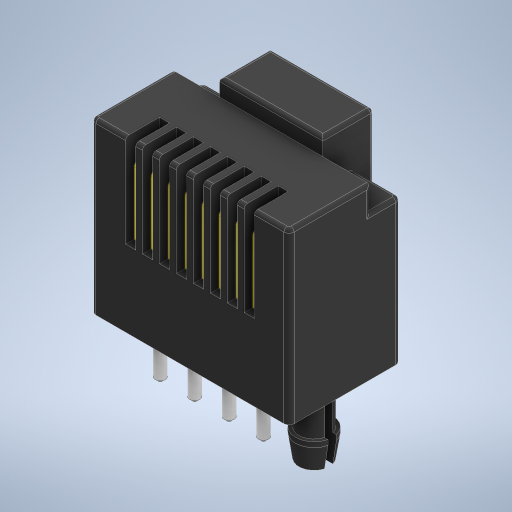
# Autodesk Inventor part: KINSUN AJP92A8813
Saved by Autodesk Inventor 2024 (Build 280153000, 153)
## iProperties
Created: 2026-08-25
Part Number: KINSUN AJP92A8813
Material: Generic
Document SubType Name: Modeling
Designer: murashkindv
Density: 1 g/cm^3
Appearance: Default
Author: murashkindv
Autodesk Inventor part; units mm, degrees
ref_plane "YZ Plane" through (0, 0, 0) normal (1, 0, 0) x (0, 1, 0)
ref_plane "XZ Plane" through (0, 0, 0) normal (0, 1, 0) x (-1, 0, 0)
ref_plane "XY Plane" through (0, 0, 0) normal (0, 0, 1) x (1, 0, 0)
sketch "Sketch6" plane through (0, 0, 0) normal (0, 1, 0) x (-1, 0, 0)
  circle A0 centre (-4.89, 0.635) radius 1.1
  circle A1 centre (4.89, -1.27) radius 1.1
  line L0 (4.89, -1.27) -> (-4.89, 0.635) construction
  line L1 (3.048, 0) -> (0, 0) construction
  line L2 (5.99, -1.52) -> (3.79, -1.52)
  line L3 (3.79, -1.52) -> (3.79, -1.02) construction
  line L4 (3.79, -1.02) -> (5.99, -1.02)
  line L5 (5.99, -1.02) -> (5.99, -1.52) construction
  line L6 (5.99, -1.52) -> (3.79, -1.02) construction
  line L7 (3.79, -1.52) -> (5.99, -1.02) construction
  line L8 (-5.99, 0.385) -> (-3.79, 0.385)
  line L9 (-3.79, 0.385) -> (-3.79, 0.885) construction
  line L10 (-3.79, 0.885) -> (-5.99, 0.885)
  line L11 (-5.99, 0.885) -> (-5.99, 0.385) construction
  line L12 (-5.99, 0.385) -> (-3.79, 0.885) construction
  line L13 (-3.79, 0.385) -> (-5.99, 0.885) construction
  point P0 (0, -0.3175)
  point P1 (-3.79, 0.635)
  point P2 (-4.64, -0.4362)
  point P3 (-5.14, -0.4362)
  point P4 (-5.99, 0.635)
  point P5 (3.79, -1.27)
  point P6 (4.64, -0.1988)
  point P7 (5.99, -1.27)
  point P8 (5.14, -2.3412)
  point P9 (-5.9612, 0.885)
  point P10 (-3.8188, 0.885)
  point P11 (-5.9612, 0.385)
  point P12 (-3.8188, 0.385)
  point P13 (5.9612, -1.02)
  point P14 (5.9612, -1.52)
  point P15 (3.8188, -1.02)
  point P16 (3.8188, -1.52)
  dimension "d77" = 2.2
  dimension "d78" = 9.78
  dimension "d89" = 1.27
  dimension "d90" = 0.635
  dimension "d160" = 0.5
  constraints: 28 end point, 6 parallel, 5 midpoint, 3 horizontal, 2 centre point, 2 perpendicular, 1 coincident, 1 equal radius, 1 horizontal alignment, 1 tangent, 1 vertical alignment, 1 other
  measures "d77" diameter of A1
  measures "d78" horizontal distance of L0.end L0.start
  measures "d89" vertical distance of L1.end L0.start
  measures "d90" vertical distance of L1.end L0.end
  measures "d160" distance between parallel lines of L2 L4
sketch "Sketch7" plane through (0, 0, 0) normal (0, 1, 0) x (-1, 0, 0)
  circle A0 centre (2.54, -1.27) radius 0.3
  circle A1 centre (3.556, 1.27) radius 0.3
  line L0 (2.54, -1.27) -> (3.556, 1.27) construction
  line L1 (3.048, 0) -> (0, 0) construction
  circle A2 centre (0.508, -1.27) radius 0.3
  circle A3 centre (1.524, 1.27) radius 0.3
  circle A4 centre (-1.524, -1.27) radius 0.3
  circle A5 centre (-0.508, 1.27) radius 0.3
  circle A6 centre (-3.556, -1.27) radius 0.3
  circle A7 centre (-2.54, 1.27) radius 0.3
  line L2 (-2.54, 1.27) -> (2.54, -1.27) construction
  dimension "d95" = 0.6
  dimension "d97" = 1.016
  dimension "d98" = 2.032
  dimension "d99" = 7.112
  dimension "d101" = 1.27
  constraints: 8 centre point, 6 end point, 2 horizontal, 2 midpoint, 1 coincident, 1 equal radius, 1 horizontal alignment, 12 other
  measures "d95" diameter of A0
  measures "d97" horizontal distance of L0.end L2.end
  measures "d98" distance of L2.end A2.centre
  measures "d99" horizontal distance of A6.centre L0.end
  measures "d101" vertical distance of point (0, 0) L2.end
sketch "Sketch8" plane through (0, 0, 0) normal (0, 1, 0) x (-1, 0, 0)
  line L0 (5.55, -3.525) -> (-5.55, -3.525)
  line L1 (-5.85, -3.225) -> (-5.85, 2.775)
  line L2 (-5.55, 3.075) -> (5.55, 3.075)
  line L3 (5.85, 2.775) -> (5.85, -3.225)
  arc A0 (5.55, -3.525) -> (5.85, -3.225) centre (5.55, -3.225) ccw
  arc A1 (5.85, 2.775) -> (5.55, 3.075) centre (5.55, 2.775) ccw
  arc A2 (-5.55, 3.075) -> (-5.85, 2.775) centre (-5.55, 2.775) ccw
  arc A3 (-5.85, -3.225) -> (-5.55, -3.525) centre (-5.55, -3.225) ccw
  line L4 (3.05, -3.525) -> (-3.05, -3.525)
  line L5 (-3.05, -3.525) -> (-3.05, -4.725)
  line L6 (-3.05, -4.725) -> (3.05, -4.725)
  line L7 (3.05, -4.725) -> (3.05, -3.525)
  point P0 (0, 0)
  point P1 (5.85, -3.525)
  point P2 (-5.85, 3.075)
  point P3 (5.85, 3.075)
  point P4 (0, -3.525)
  point P5 (0, -4.725)
  point P6 (0, -3.525)
  dimension "d102" = 3.525
  dimension "d103" = 6.6
  dimension "d104" = 11.7
  dimension "d105" = 0.3
  dimension "d106" = 6.1
  dimension "d107" = 1.2
  constraints: 16 end point, 8 point on circle, 8 tangent, 7 point on line, 4 centre point, 4 parallel, 3 equal radius, 3 midpoint, 3 vertical alignment, 2 horizontal, 2 perpendicular
  measures "d102" distance from line of point (0, 0) L0
  measures "d103" distance of point (5.85, 3.075) point (5.85, -3.525)
  measures "d104" distance of point (-5.85, 3.075) point (5.85, 3.075)
  measures "d105" radius of A0
  measures "d106" distance of L5.end L6.end
  measures "d107" distance of L6.end L4.start
extrude "Extrusion5" add sketch "Sketch8" along normal blind 10
sketch "Sketch13" plane through (0, 10, 0) normal (0, 1, 0) x (1, 0, 0)
  line L0 (5.55, 3.525) -> (3.05, 3.525) projected
  line L1 (3.05, 3.525) -> (3.05, 4.725) projected
  line L2 (3.05, 4.725) -> (-3.05, 4.725) projected
  line L3 (-3.05, 4.725) -> (-3.05, 3.525) projected
  line L4 (-3.05, 3.525) -> (-5.55, 3.525) projected
  arc A0 (-5.55, 3.525) -> (-5.85, 3.225) centre (-5.55, 3.225) ccw projected
  line L5 (-5.85, 3.225) -> (-5.85, -2.775) projected
  arc A1 (-5.85, -2.775) -> (-5.55, -3.075) centre (-5.55, -2.775) ccw projected
  line L6 (-5.55, -3.075) -> (5.55, -3.075) projected
  arc A2 (5.55, -3.075) -> (5.85, -2.775) centre (5.55, -2.775) ccw projected
  line L7 (5.85, -2.775) -> (5.85, 3.225) projected
  arc A3 (5.85, 3.225) -> (5.55, 3.525) centre (5.55, 3.225) ccw projected
  line L8 (-3.05, 4.725) -> (3.05, 4.725)
  line L9 (3.05, 4.725) -> (3.05, 1.725)
  line L10 (3.05, 1.725) -> (-3.05, 1.725)
  line L11 (-3.05, 1.725) -> (-3.05, 4.725)
  point P0 (0, 0)
  dimension "d161" = 3
  constraints: 8 end point, 2 parallel, 1 collinear, 1 horizontal, 1 perpendicular
  measures "d161" distance between parallel lines of L2 L10
extrude "Extrusion12" add sketch "Sketch13" along normal blind 1 contours L9 L10 L11 L3 L2 L1
sketch "Sketch9" plane through (0, 10, 0) normal (0, 1, 0) x (1, 0, 0)
  line L0 (5.55, 3.525) -> (3.05, 3.525) projected
  line L1 (-3.05, 3.525) -> (-5.55, 3.525) projected
  arc A0 (-5.55, 3.525) -> (-5.85, 3.225) centre (-5.55, 3.225) ccw projected
  line L2 (-5.85, 3.225) -> (-5.85, -2.775) projected
  arc A1 (-5.85, -2.775) -> (-5.55, -3.075) centre (-5.55, -2.775) ccw projected
  line L3 (-5.55, -3.075) -> (5.55, -3.075) projected
  arc A2 (5.55, -3.075) -> (5.85, -2.775) centre (5.55, -2.775) ccw projected
  line L4 (5.85, -2.775) -> (5.85, 3.225) projected
  arc A3 (5.85, 3.225) -> (5.55, 3.525) centre (5.55, 3.225) ccw projected
  line L5 (-3.05, 4.725) -> (3.05, 4.725)
  line L6 (3.05, 4.725) -> (3.05, 1.725)
  line L7 (3.05, 1.725) -> (-3.05, 1.725)
  line L8 (-3.05, 1.725) -> (-3.05, 4.725)
  line L9 (3.05, 3.525) -> (3.05, 4.725) projected
  line L10 (-3.05, 1.725) -> (-5.85, 1.725)
  line L11 (3.05, 1.725) -> (5.85, 1.725)
  line L12 (-3.05, 1.725) -> (-3.05, 3.525) projected
  line L13 (3.05, 3.525) -> (3.05, 1.725) projected
  line L14 (3.05, 1.725) -> (-3.05, 1.725) projected
  point P0 (0, 0)
  dimension "d110" = 3
  constraints: 12 end point, 3 point on line, 2 parallel, 2 perpendicular, 1 collinear, 1 horizontal
  measures "d110" distance of L7.end L5.start
extrude "Extrusion6" cut sketch "Sketch9" against normal blind 1.5 contours A3 L4 L11 L6 L0 | L10 L2 A0 L1 L8
extrude "Extrusion7" add sketch "Sketch6" against normal blind 3.3 contours L10 A0 | A0 L8 | L4 A1 | A1 L2
chamfer "Chamfer2" distance 0.2 distance2 1.3 2 edges at (-4.89, -3.3, -0.17) (-4.89, -3.3, -2.37) measured on face at (-5.1664, -3.3, -0.8624) measured on face at (-4.7895, -3.3, -1.8628)
chamfer "Chamfer3" distance 0.2 distance2 1.3 2 edges at (4.89, -3.3, -0.465) (4.89, -3.3, 1.735) measured on face at (5.1, -3.3, 0.1677) measured on face at (4.6136, -3.3, 1.0426)
sketch "Sketch10" plane through (0, 0, 0) normal (0, -1, 0) x (1, 0, 0)
  circle A0 centre (-4.89, -1.25) radius 0.9
  circle A1 centre (4.89, 0.635) radius 0.9
  line L0 (4.89, 0.635) -> (-4.89, -1.25) construction
  circle A2 centre (-4.89, -1.25) radius 1.3
  circle A3 centre (4.89, 0.635) radius 1.3
  point P0 (0, 0)
  point P1 (0, -0.3075)
  dimension "d121" = 1.8
  dimension "d122" = 9.78
  dimension "d125" = 1.25
  dimension "d126" = 0.635
  dimension "d127" = 2.6
  constraints: 4 centre point, 3 coincident, 2 end point, 2 equal radius, 1 midpoint, 1 vertical alignment
  measures "d121" diameter of A1
  measures "d122" horizontal distance of L0.end L0.start
  measures "d125" vertical distance of A0.centre point (0, 0)
  measures "d126" vertical distance of point (0, 0) L0.start
  measures "d127" diameter of A3
extrude "Extrusion8" cut sketch "Sketch10" along normal blind 1.7
extrude "Extrusion9" add sketch "Sketch7" against normal blind 3.25 separate body
chamfer "Chamfer4" distance 0.2 angle 45 8 edges at (-1.224, -3.25, 1.27) (-3.256, -3.25, 1.27) (0.808, -3.25, 1.27) (2.84, -3.25, 1.27) (3.856, -3.25, -1.27) (1.824, -3.25, -1.27) (-0.208, -3.25, -1.27) (-2.24, -3.25, -1.27)
sketch "Sketch11" plane through (0, 10, 0) normal (0, 1, 0) x (1, 0, 0)
  line L0 (5.85, 1.725) -> (3.05, 1.725) projected
  line L1 (-3.05, 1.725) -> (-5.85, 1.725) projected
  line L2 (-5.85, 1.725) -> (-5.85, -2.775) projected
  arc A0 (-5.85, -2.775) -> (-5.55, -3.075) centre (-5.55, -2.775) ccw projected
  line L3 (-5.55, -3.075) -> (5.55, -3.075) projected
  arc A1 (5.55, -3.075) -> (5.85, -2.775) centre (5.55, -2.775) ccw projected
  line L4 (5.85, -2.775) -> (5.85, 1.725) projected
  line L5 (-3.8, -1.075) -> (-3.2, -1.075)
  line L6 (-3.2, -1.075) -> (-3.2, -3.075)
  line L7 (-3.2, -3.075) -> (-3.8, -3.075)
  line L8 (-3.8, -3.075) -> (-3.8, -1.075)
  line L9 (-5.55, -3.075) -> (5.55, -3.075) projected
  line L10 (-2.8, -3.075) -> (-2.8, -1.075)
  line L11 (-2.8, -1.075) -> (-2.2, -1.075)
  line L12 (-2.2, -3.075) -> (-2.8, -3.075)
  line L13 (-2.2, -1.075) -> (-2.2, -3.075)
  line L14 (-1.8, -3.075) -> (-1.8, -1.075)
  line L15 (-1.8, -1.075) -> (-1.2, -1.075)
  line L16 (-1.2, -3.075) -> (-1.8, -3.075)
  line L17 (-1.2, -1.075) -> (-1.2, -3.075)
  line L18 (-0.8, -3.075) -> (-0.8, -1.075)
  line L19 (-0.8, -1.075) -> (-0.2, -1.075)
  line L20 (-0.2, -3.075) -> (-0.8, -3.075)
  line L21 (-0.2, -1.075) -> (-0.2, -3.075)
  line L22 (0.2, -3.075) -> (0.2, -1.075)
  line L23 (0.2, -1.075) -> (0.8, -1.075)
  line L24 (0.8, -3.075) -> (0.2, -3.075)
  line L25 (0.8, -1.075) -> (0.8, -3.075)
  line L26 (1.2, -3.075) -> (1.2, -1.075)
  line L27 (1.2, -1.075) -> (1.8, -1.075)
  line L28 (1.8, -3.075) -> (1.2, -3.075)
  line L29 (1.8, -1.075) -> (1.8, -3.075)
  line L30 (2.2, -3.075) -> (2.2, -1.075)
  line L31 (2.2, -1.075) -> (2.8, -1.075)
  line L32 (2.8, -3.075) -> (2.2, -3.075)
  line L33 (2.8, -1.075) -> (2.8, -3.075)
  line L34 (3.2, -3.075) -> (3.2, -1.075)
  line L35 (3.2, -1.075) -> (3.8, -1.075)
  line L36 (3.8, -3.075) -> (3.2, -3.075)
  line L37 (3.8, -1.075) -> (3.8, -3.075)
  line L38 (-3.8, -2.075) -> (3.8, -2.075) construction
  line L39 (3.05, 1.725) -> (-3.05, 1.725) projected
  point P0 (0, 0)
  point P1 (0, -2.075)
  dimension "d135" = 0.6
  dimension "d138" = 1
  dimension "d143" = 7.6
  dimension "d144" = 2
  constraints: 66 end point, 3 midpoint, 2 horizontal, 2 parallel, 1 collinear, 1 perpendicular, 1 point on line, 1 vertical alignment, 56 other
  measures "d135" distance of L5.start L5.end
  measures "d138" distance of L5.start L10.end
  measures "d143" distance between parallel lines of L37 L8
  measures "d144" distance of L7.end L5.start
extrude "Extrusion10" cut sketch "Sketch11" against normal blind 5.5 contours L3 L34 L35 L37 | L3 L30 L31 L33 | L8 L5 L6 L3 | L3 L26 L27 L29 | L10 L11 L13 L3 | L3 L22 L23 L25 | L14 L15 L17 L3 | L3 L18 L19 L21 bodies 1
sketch "Sketch12" plane through (0, 4.5, 0) normal (0, 1, 0) x (1, 0, 0)
  line L0 (-3.8, -3.075) -> (-3.8, -1.075) projected
  line L1 (-3.2, -3.075) -> (-3.8, -3.075) projected
  line L2 (-3.2, -1.075) -> (-3.2, -3.075) projected
  line L3 (-3.8, -1.075) -> (-3.2, -1.075) projected
  line L4 (-2.8, -3.075) -> (-2.8, -1.075) projected
  line L5 (-2.2, -3.075) -> (-2.8, -3.075) projected
  line L6 (-2.2, -1.075) -> (-2.2, -3.075) projected
  line L7 (-2.8, -1.075) -> (-2.2, -1.075) projected
  line L8 (-1.8, -3.075) -> (-1.8, -1.075) projected
  line L9 (-1.2, -3.075) -> (-1.8, -3.075) projected
  line L10 (-1.2, -1.075) -> (-1.2, -3.075) projected
  line L11 (-1.8, -1.075) -> (-1.2, -1.075) projected
  line L12 (-0.8, -3.075) -> (-0.8, -1.075) projected
  line L13 (-0.2, -3.075) -> (-0.8, -3.075) projected
  line L14 (-0.2, -1.075) -> (-0.2, -3.075) projected
  line L15 (-0.8, -1.075) -> (-0.2, -1.075) projected
  line L16 (0.2, -3.075) -> (0.2, -1.075) projected
  line L17 (0.8, -3.075) -> (0.2, -3.075) projected
  line L18 (0.8, -1.075) -> (0.8, -3.075) projected
  line L19 (0.2, -1.075) -> (0.8, -1.075) projected
  line L20 (1.2, -3.075) -> (1.2, -1.075) projected
  line L21 (1.8, -3.075) -> (1.2, -3.075) projected
  line L22 (1.8, -1.075) -> (1.8, -3.075) projected
  line L23 (1.2, -1.075) -> (1.8, -1.075) projected
  line L24 (2.2, -3.075) -> (2.2, -1.075) projected
  line L25 (2.8, -3.075) -> (2.2, -3.075) projected
  line L26 (2.8, -1.075) -> (2.8, -3.075) projected
  line L27 (2.2, -1.075) -> (2.8, -1.075) projected
  line L28 (3.2, -3.075) -> (3.2, -1.075) projected
  line L29 (3.8, -3.075) -> (3.2, -3.075) projected
  line L30 (3.8, -1.075) -> (3.8, -3.075) projected
  line L31 (3.2, -1.075) -> (3.8, -1.075) projected
  line L32 (-3.8, -1.075) -> (-3.2, -1.075)
  line L33 (-3.2, -1.075) -> (-3.2, -2.575)
  line L34 (-3.2, -2.575) -> (-3.8, -2.575)
  line L35 (-3.8, -2.575) -> (-3.8, -1.075)
  line L36 (-2.2, -1.075) -> (-2.2, -2.575)
  line L37 (-2.8, -2.575) -> (-2.8, -1.075)
  line L38 (-2.2, -2.575) -> (-2.8, -2.575)
  line L39 (-2.8, -1.075) -> (-2.2, -1.075)
  line L40 (-1.2, -1.075) -> (-1.2, -2.575)
  line L41 (-1.8, -2.575) -> (-1.8, -1.075)
  line L42 (-1.2, -2.575) -> (-1.8, -2.575)
  line L43 (-1.8, -1.075) -> (-1.2, -1.075)
  line L44 (-0.2, -1.075) -> (-0.2, -2.575)
  line L45 (-0.8, -2.575) -> (-0.8, -1.075)
  line L46 (-0.2, -2.575) -> (-0.8, -2.575)
  line L47 (-0.8, -1.075) -> (-0.2, -1.075)
  line L48 (0.8, -1.075) -> (0.8, -2.575)
  line L49 (0.2, -2.575) -> (0.2, -1.075)
  line L50 (0.8, -2.575) -> (0.2, -2.575)
  line L51 (0.2, -1.075) -> (0.8, -1.075)
  line L52 (1.8, -1.075) -> (1.8, -2.575)
  line L53 (1.2, -2.575) -> (1.2, -1.075)
  line L54 (1.8, -2.575) -> (1.2, -2.575)
  line L55 (1.2, -1.075) -> (1.8, -1.075)
  line L56 (2.8, -1.075) -> (2.8, -2.575)
  line L57 (2.2, -2.575) -> (2.2, -1.075)
  line L58 (2.8, -2.575) -> (2.2, -2.575)
  line L59 (2.2, -1.075) -> (2.8, -1.075)
  line L60 (3.8, -1.075) -> (3.8, -2.575)
  line L61 (3.2, -2.575) -> (3.2, -1.075)
  line L62 (3.8, -2.575) -> (3.2, -2.575)
  line L63 (3.2, -1.075) -> (3.8, -1.075)
  point P0 (0, 0)
  dimension "d150" = 1
  dimension "d155" = 0.5
  constraints: 64 end point, 2 horizontal, 2 parallel, 1 perpendicular, 1 point on line, 63 other
  measures "d150" distance of L0.end L37.end
  measures "d155" distance between parallel lines of L1 L34
extrude "Extrusion11" add sketch "Sketch12" along normal blind 4 separate body contours L0 L3 L2 L34 | L4 L7 L6 L38 | L8 L11 L10 L42 | L12 L15 L14 L46 | L16 L19 L18 L50 | L20 L23 L22 L54 | L24 L27 L26 L58 | L28 L31 L30 L62
fillet "Fillet4" radius 0.3 8 edges at (-3.5, 8.5, 2.575) (-2.5, 8.5, 2.575) (-1.5, 8.5, 2.575) (-0.5, 8.5, 2.575) (0.5, 8.5, 2.575) (1.5, 8.5, 2.575) (2.5, 8.5, 2.575) (3.5, 8.5, 2.575)
fillet "Fillet5" radius 0.2 26 edges at (3.05, 5.5, -4.725) (3.05, 11, -3.225) (0, 11, -4.725) (-3.05, 11, -3.225) (0, 11, -1.725) (-5.7621, 10, 2.9871) (-4.675, 10, 3.075) (-5.85, 10, 0.525) (5.7621, 10, 2.9871) (4.675, 10, 3.075) (5.85, 10, 0.525) (-5.7621, 8.5, -3.4371) (-5.85, 8.5, -2.475) (-4.3, 8.5, -3.525) (5.7621, 8.5, -3.4371) (5.85, 8.5, -2.475) (4.3, 8.5, -3.525) (5.85, 9.25, -1.725) (-5.85, 9.25, -1.725) (-3, 10, 3.075) (-2, 10, 3.075) (-1, 10, 3.075) (0, 10, 3.075) (1, 10, 3.075) (2, 10, 3.075) (3, 10, 3.075)
body "Solid2"
body "Solid3"
body "Solid4"
